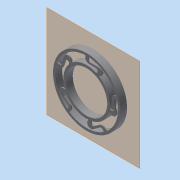
# Autodesk Inventor part: 01_Autofocus_CCTV12mm_spring_1
Saved by Autodesk Inventor 2019.4 (Build 234330000, 330)
## iProperties
Created: 2020-10-23
Part Number: 01_Autofocus_CCTV12mm_spring_1
Material: Generic
Document SubType Name: Modeling
Designer: diederichbenedict
Density: 1 g/cm^3
Appearance: Default
Author: diederichbenedict
Autodesk Inventor part; units mm, degrees
ref_plane "YZ Plane" through (0, 0, 0) normal (1, 0, 0) x (0, 1, 0)
ref_plane "XZ Plane" through (0, 0, 0) normal (0, 1, 0) x (-1, 0, 0)
ref_plane "XY Plane" through (0, 0, 0) normal (0, 0, 1) x (1, 0, 0)
ref_plane "Work Plane1" through (-22.2084, -34.255, 31.6599) normal (0, 0, 1) x (-1, 0, 0)
sketch "Sketch1" plane through (-22.2084, -34.255, 31.6599) normal (0, 0, 1) x (-1, 0, 0)
  circle A0 centre (0, 0) radius 8.175
  circle A1 centre (0, 0) radius 8.975
  circle A2 centre (0, 0) radius 12.025
  circle A3 centre (0, 0) radius 8.1117 projected
  circle A4 centre (0, 0) radius 14.025
  point P0 (-22.2084, -34.255)
  dimension "d0" = 16.35
  dimension "d1" = 0.8
  dimension "d35" = 3.05
  dimension "d36" = 2
  constraints: 4 centre point, 1 coincident
  measures "d0" diameter of A0
  measures "d1" radial gap between concentric circles of A0 A1
  measures "d35" radial gap between concentric circles of A1 A2
  measures "d36" radial gap between concentric circles of A2 A4
extrude "Extrusion1" add sketch "Sketch1" along normal blind 2 contours A1 | A4
sketch "Sketch2" plane through (-22.2084, -34.255, 33.6599) normal (0, 0, 1) x (1, 0, 0)
  circle A0 centre (0, 0) radius 8.175 construction
  circle A1 centre (0, 0) radius 8.975 construction
  circle A2 centre (0, 0) radius 9.25 construction
  line L0 (0.1042, 9.2494) -> (0.1042, 8.4994) construction
  circle A3 centre (0, 0) radius 8.975 construction
  line L1 (3.5405, 9.5401) -> (0.126, 9.5401) construction
  line L2 (0.126, 9.5401) -> (0.126, 8.9741) construction
  line L3 (3.5405, 9.5401) -> (0.9587, 9.5401)
  line L4 (0.6463, 8.9696) -> (0.6463, 8.9517)
  line L5 (4.6302, 10.1689) -> (2.2495, 10.1689)
  line L6 (0.4, 12.0183) -> (0.4, 9.2413)
  arc A4 (0.6463, 8.9517) -> (0.6463, 8.9517) centre (1.4268, -3.3321) ccw
  line L7 (-21.2717, 34.255) -> (29.4551, 34.255) projected
  arc A5 (4.6302, 7.6884) -> (4.6302, 10.1689) centre (4.6302, 8.9286) ccw
  arc A6 (3.5405, 8.2472) -> (3.5405, 9.5401) centre (3.5405, 8.8936) ccw
  arc A7 (4.6302, 7.6884) -> (3.5405, 8.2472) centre (0, 0) ccw
  arc A8 (0.4, 9.2413) -> (-0.0924, 9.2495) centre (0, 0) ccw
  arc A9 (4.6302, 7.6884) -> (3.1121, 8.4181) centre (0, 0) ccw construction
  arc A10 (0.4, 12.0183) -> (2.2495, 10.1689) centre (2.2495, 12.0183) ccw
  line L8 (22.2084, -23.681) -> (22.2084, 43.911) projected
  arc A11 (-0.8047, 11.3035) -> (0.9587, 9.5401) centre (0.9587, 11.3035) ccw
  line L9 (-0.8047, 11.998) -> (-0.8047, 11.3035)
  circle A12 centre (0, 0) radius 12.025 projected
  arc A13 (0.4, 12.0183) -> (-0.8047, 11.998) centre (0, 0) ccw
  point P0 (22.2084, 34.255)
  point P1 (-2.5828, 8.8821)
  point P2 (-2.5828, 8.8821)
  point P3 (0.6463, 8.9517)
  point P4 (4.3208, 9.5401)
  dimension "d31" = 0.4
  constraints: 24 point on circle, 16 end point, 9 centre point, 6 tangent, 4 coincident, 2 horizontal, 2 parallel, 2 vertical, 1 concentric, 1 perpendicular, 1 point on line, 23 other
  measures "d31" distance from line of A0.centre L6
extrude "Extrusion2" add sketch "Sketch2" against normal blind 0.3 contours L3 A11 L6 A10 L5 A5 A4 A6 | A4 A5 A7 A6 | A11 L9 A12 L6
pattern_circular "Circular Pattern1" count 5 over 360 about axis through (-22.2084, -34.255, 31.6599) along (0, 0, 1) of "Extrusion2"
equation "\"d31\" = d_1"
equation "\"d_1\" = 0.4"
body "Solid1"
